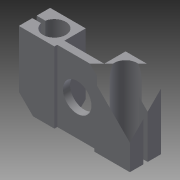
# Autodesk Inventor part: XCarriageV2
Saved by Autodesk Inventor 2015 (Build 190159000, 159)
## iProperties
Created: 2014-08-17
Part Number: XCarriageV2
Material: Generic
Document SubType Name: Modeling
Designer: Jack
Density: 1 g/cm^3
Appearance: Default
Author: Jack
Autodesk Inventor part; units mm, degrees
ref_plane "YZ Plane" through (0, 0, 0) normal (1, 0, 0) x (0, 1, 0)
ref_plane "XZ Plane" through (0, 0, 0) normal (0, 1, 0) x (-1, 0, 0)
ref_plane "XY Plane" through (0, 0, 0) normal (0, 0, 1) x (1, 0, 0)
sketch "Sketch1" plane through (0, 0, 0) normal (0, 0, 1) x (1, 0, 0)
  arc A0 (-7.8581, -1.5) -> (-7.8581, 1.5) centre (0, 0) ccw
  arc A1 (47.8581, 1.5) -> (47.8581, -1.5) centre (40, 0) ccw
  line L0 (11, -4) -> (11, 11)
  line L1 (11, 11) -> (-14, 11)
  line L2 (-14, 11) -> (-14, 1.5)
  line L3 (-14, 1.5) -> (-7.8581, 1.5)
  line L4 (11, -4) -> (29, -4)
  line L5 (29, -4) -> (29, 11)
  line L6 (29, 11) -> (54, 11)
  line L7 (54, 11) -> (54, 1.5)
  line L8 (54, 1.5) -> (47.8581, 1.5)
  line L9 (-7.8581, -1.5) -> (-14, -1.5)
  line L10 (-14, -1.5) -> (-14, -11)
  line L11 (-14, -11) -> (11, -11)
  line L12 (11, -11) -> (11, -9)
  line L13 (11, -9) -> (29, -9)
  line L14 (29, -9) -> (29, -11)
  line L15 (29, -11) -> (54, -11)
  line L16 (54, -11) -> (54, -1.5)
  line L17 (54, -1.5) -> (47.8581, -1.5)
  dimension "d0" = 16
  dimension "d1" = 16
  dimension "d2" = 40
  dimension "d3" = 1.5
  dimension "d4" = 1.5
  dimension "d5" = 14
  dimension "d6" = 14
  dimension "d7" = 5
  dimension "d8" = 11
  dimension "d9" = 11
  dimension "d10" = 15
  dimension "d11" = 11
  dimension "d12" = 11
  constraints: 36 end point, 13 perpendicular, 4 point on circle, 4 vertical alignment, 3 horizontal, 3 horizontal alignment, 3 point on line, 2 centre point, 1 coincident, 1 vertical
  measures "d0" diameter of A0
  measures "d1" diameter of A1
  measures "d2" distance of point (0, 0) A1.centre
  measures "d3" distance from line of A1.centre L17
  measures "d4" distance from line of A1.centre L8
  measures "d5" distance from line of A1.centre L7
  measures "d6" distance from line of L2 point (0, 0)
  measures "d7" distance between parallel lines of L4 L13
  measures "d8" distance from line of point (0, 0) L11
  measures "d9" distance from line of L1 point (0, 0)
  measures "d10" distance between parallel lines of L1 L4
  measures "d11" distance from line of point (0, 0) L12
  measures "d12" distance from line of L5 A1.centre
extrude "Extrusion1" add sketch "Sketch1" along normal blind 50
sketch "Sketch2" plane through (11, -4, 0) normal (0, 1, 0) x (1, 0, 0)
  line L0 (18, -50) -> (0, -50) projected
  line L1 (18, 0) -> (18, -50) projected
  circle A0 centre (9, -25) radius 9
  point P0 (-11, 0)
  dimension "d15" = 18
  dimension "d16" = 25
  dimension "d17" = 9
  constraints: 1 centre point
  measures "d15" diameter of A0
  measures "d16" distance from line of L0 A0.centre
  measures "d17" distance from line of L1 A0.centre
extrude "Extrusion2" cut sketch "Sketch2" against normal up to surface (5 mm away)
body "Solid1"
